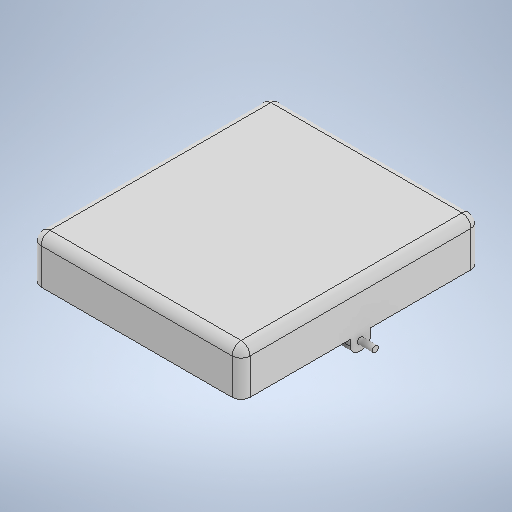
# Autodesk Inventor part: base_link
Saved by Autodesk Inventor 2025.2 (Build 292293000, 293)
## iProperties
Created: 2025-11-14
Part Number: base_link
Material: Genérico
Document SubType Name: Modeling
Designer: igles
Density: 1 g/cm^3
Appearance: Valor por defecto
Author: igles
Autodesk Inventor part; units mm, degrees
ref_plane "YZ Plane" through (0, 0, 0) normal (1, 0, 0) x (0, 1, 0)
ref_plane "XZ Plane" through (0, 0, 0) normal (0, 1, 0) x (-1, 0, 0)
ref_plane "XY Plane" through (0, 0, 0) normal (0, 0, 1) x (1, 0, 0)
sketch "Boceto1" plane through (0, 0, 0) normal (0, 1, 0) x (-1, 0, 0)
  line L0 (-350, 400) -> (350, 400)
  line L1 (350, 400) -> (350, -400)
  line L2 (350, -400) -> (-350, -400)
  line L3 (-350, -400) -> (-350, 400)
  line L4 (-350, 400) -> (350, -400) construction
  line L5 (350, 400) -> (-350, -400) construction
  point P0 (0, 0)
  dimension "d0" = 700
  dimension "d1" = 800
  constraints: 12 end point, 2 midpoint, 2 parallel, 1 horizontal, 1 perpendicular
  measures "d0" distance of L1.end L2.end
  measures "d1" distance of L0.end L1.end
extrude "Extrusión1" add sketch "Boceto1" along normal blind 150
fillet "Empalme1" radius 30 8 edges at (350, 150, 0) (0, 150, -400) (0, 150, 400) (-350, 150, 0) (-350, 75, 400) (350, 75, 400) (350, 75, -400) (-350, 75, -400)
sketch "Boceto2" plane through (0, 0, 0) normal (0, -1, 0) x (1, 0, 0)
  line L0 (-350, -370) -> (-350, 370) projected
  line L1 (-142.3817, -33.9222) -> (-350, -33.9222)
  line L2 (-350, -33.9222) -> (-350, 33.9222)
  line L3 (-350, 33.9222) -> (-142.3817, 33.9222)
  line L4 (-142.3817, 33.9222) -> (-142.3817, -33.9222)
  line L5 (-142.3817, -33.9222) -> (-350, 33.9222) construction
  line L6 (-350, -33.9222) -> (-142.3817, 33.9222) construction
  line L7 (0, 160.6517) -> (0, -134.4555)
  line L8 (142.3817, -33.9222) -> (350, -33.9222)
  line L9 (350, -33.9222) -> (350, 33.9222)
  line L10 (350, 33.9222) -> (142.3817, 33.9222)
  line L11 (142.3817, 33.9222) -> (142.3817, -33.9222)
  line L12 (142.3817, -33.9222) -> (350, 33.9222) construction
  line L13 (350, -33.9222) -> (142.3817, 33.9222) construction
  point P0 (0, 0)
  point P1 (-246.1908, 0)
  point P2 (246.1908, 0)
  constraints: 26 end point, 5 symmetric about line, 2 midpoint, 2 parallel, 1 horizontal, 1 perpendicular, 1 point on line, 1 vertical
extrude "Extrusión2" add sketch "Boceto2" along normal blind 50
fillet "Empalme2" radius 30 4 edges at (-246.1908, -50, 33.9222) (-246.1908, -50, -33.9222) (246.1908, -50, 33.9222) (246.1908, -50, -33.9222)
sketch "Boceto3" plane through (-350, 0, 370) normal (-1, 0, 0) x (0, 0, 1)
  circle A0 centre (-370, -20) radius 10.25
  point P0 (-370, 0)
  dimension "d8" = 20.5
  constraints: 1 centre point
  measures "d8" diameter of A0
extrude "Extrusión3" add sketch "Boceto3" along normal blind 50
sketch "Boceto4" plane through (350, 0, -370) normal (1, 0, 0) x (0, 0, -1)
  circle A0 centre (-370, -20) radius 10.25 projected
  circle A1 centre (-370, -20) radius 10.25
  point P0 (-370, 0)
  constraints: 1 centre point, 1 coincident
extrude "Extrusión4" add sketch "Boceto4" along normal blind 50
